bart pro xl bottom z rod guide v2 (Autodesk Fusion 360 design; units mm, degrees)
Autodesk Fusion 360 part; units mm, degrees
sketch "Sketch3" plane through (0, 0, 0) normal (0, 0, 1) x (1, 0, 0)
  line L0 (0, 45) -> (10, 45) construction
  line L1 (10, 45) -> (16, 45) construction
  line L2 (9.5, 35) -> (9.5, 52) construction
  line L3 (-7.3524, 60.5) -> (6.5625, 60.5) construction
  line L4 (0, 63) -> (0, 27) construction
  line L5 (-2, 29.5) -> (5, 29.5) construction
  circle A0 centre (9.5, 45) radius 5.5 construction
  circle A1 centre (0, 60.5) radius 2 construction
  circle A2 centre (0, 29.5) radius 2 construction
  line L6 (-3, 64) -> (17, 64)
  line L7 (17, 64) -> (17, 26)
  line L8 (17, 26) -> (-3, 26)
  line L9 (-3, 26) -> (-3, 64)
  line L10 (6.5625, 60.5) -> (7, 60.5)
  line L11 (7, 60.5) -> (26.4352, 60.5) construction
  line L12 (9.5, 52) -> (9.5, 63) construction
  line L13 (9.5, 35) -> (9.5, 24) construction
  line L14 (5, 29.5) -> (7, 29.5) construction
  line L15 (7, 29.5) -> (31, 29.5) construction
  dimension "d8" = 11
  dimension "d9" = 4
  constraint horizontal L0
  constraint parallel L0 L1
  constraint perpendicular L0 L4
  constraint perpendicular L4 L5
  constraint coincident L4
  constraint coincident L3
  constraint coincident L2
  constraint coincident L0
  constraint coincident L5
  constraint perpendicular L4 L6
  constraint perpendicular L6 L7
  constraint perpendicular L4 L8
  constraint perpendicular L6 L9
  constraint parallel L3 L10
  constraint parallel L3 L11
  constraint perpendicular L11 L12
  constraint perpendicular L8 L13
  constraint perpendicular L13 L15
  constraint coincident L12
  constraint coincident L11
  constraint midpoint L13
  measures "d8" diameter of A0
  measures "d9" diameter of A1
extrude "Extrude4" add sketch "Sketch3" along normal blind 3
hole "Hole1" at (0.0867, 60.5074, 3) direction (0, 0, -1) diameter 4 end through all
hole "Hole2" at (0.0867, 29.4547, 3) direction (0, 0, -1) diameter 4 end through all
sketch "Sketch4" plane through (0, 0, 3) normal (0, 0, 1) x (-1, 0, 0)
  circle A0 centre (-0.0867, -29.4547) radius 2
  circle A1 centre (-0.0867, -60.5074) radius 2
  line L0 (3, -26) -> (-17, -26)
  line L1 (-17, -26) -> (-17, -64)
  line L2 (-17, -64) -> (3, -64)
  line L3 (3, -64) -> (3, -26)
  circle A2 centre (-9.5, -45) radius 5.25
  circle A3 centre (-9.5, -45) radius 6.25
  dimension "d18" = 10.5
  dimension "d19" = 12.5
  measures "d18" diameter of A2
  measures "d19" diameter of A3
extrude "Extrude5" add sketch "Sketch4" along normal blind 3 contours A3
hole "Hole3" at (9.3938, 60.3234, 0) direction (0, 0, 1) diameter 4 end through all
hole "Hole4" at (9.534, 29.338, 0) direction (0, 0, 1) diameter 4 end through all
